Autodesk Inventor part; units mm, degrees
(part 2 of 3)
  arc A340 (-25.1328, 93.8701) -> (-24.6328, 93.3701) centre (-24.6328, 93.8701) ccw
  arc A341 (-24.6328, 100.3701) -> (-25.1328, 99.8701) centre (-24.6328, 99.8701) ccw
  arc A342 (-10.6328, 93.3701) -> (-10.1328, 93.8701) centre (-10.6328, 93.8701) ccw
  arc A343 (-10.1328, 99.8701) -> (-10.6328, 100.3701) centre (-10.6328, 99.8701) ccw
  line L344 (-25.1328, 193.8701) -> (-25.1328, 199.8701)
  line L345 (-10.1328, 193.8701) -> (-10.1328, 199.8701)
  line L346 (-24.6328, 193.3701) -> (-10.6328, 193.3701)
  line L347 (-24.6328, 200.3701) -> (-10.6328, 200.3701)
  arc A344 (-25.1328, 193.8701) -> (-24.6328, 193.3701) centre (-24.6328, 193.8701) ccw
  arc A345 (-24.6328, 200.3701) -> (-25.1328, 199.8701) centre (-24.6328, 199.8701) ccw
  arc A346 (-10.6328, 193.3701) -> (-10.1328, 193.8701) centre (-10.6328, 193.8701) ccw
  arc A347 (-10.1328, 199.8701) -> (-10.6328, 200.3701) centre (-10.6328, 199.8701) ccw
  line L348 (-26.1328, 211.8076) -> (-26.1328, 224.8076)
  line L349 (-12.1328, 211.8076) -> (-12.1328, 224.8076)
  line L350 (-25.6328, 211.3076) -> (-12.6328, 211.3076)
  line L351 (-25.6328, 225.3076) -> (-12.6328, 225.3076)
  arc A348 (-26.1328, 211.8076) -> (-25.6328, 211.3076) centre (-25.6328, 211.8076) ccw
  arc A349 (-25.6328, 225.3076) -> (-26.1328, 224.8076) centre (-25.6328, 224.8076) ccw
  arc A350 (-12.6328, 211.3076) -> (-12.1328, 211.8076) centre (-12.6328, 211.8076) ccw
  arc A351 (-12.1328, 224.8076) -> (-12.6328, 225.3076) centre (-12.6328, 224.8076) ccw
  line L352 (-26.1328, 235.6201) -> (-26.1328, 248.6201)
  line L353 (-12.1328, 235.6201) -> (-12.1328, 248.6201)
  line L354 (-25.6328, 235.1201) -> (-12.6328, 235.1201)
  line L355 (-25.6328, 249.1201) -> (-12.6328, 249.1201)
  arc A352 (-26.1328, 235.6201) -> (-25.6328, 235.1201) centre (-25.6328, 235.6201) ccw
  arc A353 (-25.6328, 249.1201) -> (-26.1328, 248.6201) centre (-25.6328, 248.6201) ccw
  arc A354 (-12.6328, 235.1201) -> (-12.1328, 235.6201) centre (-12.6328, 235.6201) ccw
  arc A355 (-12.1328, 248.6201) -> (-12.6328, 249.1201) centre (-12.6328, 248.6201) ccw
  line L356 (-26.1328, 259.4326) -> (-26.1328, 272.4326)
  line L357 (-12.1328, 259.4326) -> (-12.1328, 272.4326)
  line L358 (-25.6328, 258.9326) -> (-12.6328, 258.9326)
  line L359 (-25.6328, 272.9326) -> (-12.6328, 272.9326)
  arc A356 (-26.1328, 259.4326) -> (-25.6328, 258.9326) centre (-25.6328, 259.4326) ccw
  arc A357 (-25.6328, 272.9326) -> (-26.1328, 272.4326) centre (-25.6328, 272.4326) ccw
  arc A358 (-12.6328, 258.9326) -> (-12.1328, 259.4326) centre (-12.6328, 259.4326) ccw
  arc A359 (-12.1328, 272.4326) -> (-12.6328, 272.9326) centre (-12.6328, 272.4326) ccw
  line L360 (-26.1328, 283.2451) -> (-26.1328, 296.2451)
  line L361 (-12.1328, 283.2451) -> (-12.1328, 296.2451)
  line L362 (-25.6328, 282.7451) -> (-12.6328, 282.7451)
  line L363 (-25.6328, 296.7451) -> (-12.6328, 296.7451)
  arc A360 (-26.1328, 283.2451) -> (-25.6328, 282.7451) centre (-25.6328, 283.2451) ccw
  arc A361 (-25.6328, 296.7451) -> (-26.1328, 296.2451) centre (-25.6328, 296.2451) ccw
  arc A362 (-12.6328, 282.7451) -> (-12.1328, 283.2451) centre (-12.6328, 283.2451) ccw
  arc A363 (-12.1328, 296.2451) -> (-12.6328, 296.7451) centre (-12.6328, 296.2451) ccw
  line L364 (-26.1328, 309.4388) -> (-26.1328, 322.4388)
  line L365 (-12.1328, 309.4388) -> (-12.1328, 322.4388)
  line L366 (-25.6328, 308.9388) -> (-12.6328, 308.9388)
  line L367 (-25.6328, 322.9388) -> (-12.6328, 322.9388)
  arc A364 (-26.1328, 309.4388) -> (-25.6328, 308.9388) centre (-25.6328, 309.4388) ccw
  arc A365 (-25.6328, 322.9388) -> (-26.1328, 322.4388) centre (-25.6328, 322.4388) ccw
  arc A366 (-12.6328, 308.9388) -> (-12.1328, 309.4388) centre (-12.6328, 309.4388) ccw
  arc A367 (-12.1328, 322.4388) -> (-12.6328, 322.9388) centre (-12.6328, 322.4388) ccw
  line L368 (-26.1328, 328.4888) -> (-26.1328, 341.4888)
  line L369 (-12.1328, 328.4888) -> (-12.1328, 341.4888)
  line L370 (-25.6328, 327.9888) -> (-12.6328, 327.9888)
  line L371 (-25.6328, 341.9888) -> (-12.6328, 341.9888)
  arc A368 (-26.1328, 328.4888) -> (-25.6328, 327.9888) centre (-25.6328, 328.4888) ccw
  arc A369 (-25.6328, 341.9888) -> (-26.1328, 341.4888) centre (-25.6328, 341.4888) ccw
  arc A370 (-12.6328, 327.9888) -> (-12.1328, 328.4888) centre (-12.6328, 328.4888) ccw
  arc A371 (-12.1328, 341.4888) -> (-12.6328, 341.9888) centre (-12.6328, 341.4888) ccw
  line L372 (-26.1328, 347.5388) -> (-26.1328, 360.5388)
  line L373 (-12.1328, 347.5388) -> (-12.1328, 360.5388)
  line L374 (-25.6328, 347.0388) -> (-12.6328, 347.0388)
  line L375 (-25.6328, 361.0388) -> (-12.6328, 361.0388)
  arc A372 (-26.1328, 347.5388) -> (-25.6328, 347.0388) centre (-25.6328, 347.5388) ccw
  arc A373 (-25.6328, 361.0388) -> (-26.1328, 360.5388) centre (-25.6328, 360.5388) ccw
  arc A374 (-12.6328, 347.0388) -> (-12.1328, 347.5388) centre (-12.6328, 347.5388) ccw
  arc A375 (-12.1328, 360.5388) -> (-12.6328, 361.0388) centre (-12.6328, 360.5388) ccw
  line L376 (-9.6078, 15.9013) -> (-9.6078, 363.5638)
  line L377 (-133.4328, 15.9013) -> (-133.4328, 363.5638)
  line L378 (-9.6078, 15.9013) -> (-133.4328, 15.9013)
  line L379 (-9.6078, 363.5638) -> (-133.4328, 363.5638)
  point P0 (-68.7393, 181.4626)
sketch "Sketch1" plane through (0, 0, 0) normal (0, 1, 0) x (-1, 0, 0)
  line L0 (0, 0) -> (144.19, 0)
  line L1 (144.19, 0) -> (144.19, -379.14)
  line L2 (144.19, -379.14) -> (0, -379.14)
  line L3 (0, -379.14) -> (0, 0)
  dimension "d0" = 144.19
  dimension "d1" = 379.14
  constraints: 8 end point, 2 parallel, 1 horizontal, 1 perpendicular
  measures "d0" distance of L1.end L2.end
  measures "d1" distance of L0.end L1.end
extrude "Extrusion1" add sketch "Sketch1" along normal blind 2
sketch "Sketch3" plane through (0, 2, 0) normal (0, 1, 0) x (1, 0, 0)
  line L0 (-144.19, 0) -> (0, 0) projected
  line L1 (-144.19, 379.14) -> (-144.19, 0) projected
  line L2 (-131.665, 13.025) -> (-131.665, 26.025)
  line L3 (-117.665, 13.025) -> (-117.665, 26.025)
  line L4 (-131.165, 12.525) -> (-118.165, 12.525)
  line L5 (-131.165, 26.525) -> (-118.165, 26.525)
  arc A0 (-131.665, 13.025) -> (-131.165, 12.525) centre (-131.165, 13.025) ccw
  arc A1 (-131.165, 26.525) -> (-131.665, 26.025) centre (-131.165, 26.025) ccw
  arc A2 (-118.165, 12.525) -> (-117.665, 13.025) centre (-118.165, 13.025) ccw
  arc A3 (-117.665, 26.025) -> (-118.165, 26.525) centre (-118.165, 26.025) ccw
  line L6 (-131.665, 51.125) -> (-131.665, 64.125)
  line L7 (-117.665, 51.125) -> (-117.665, 64.125)
  line L8 (-131.165, 50.625) -> (-118.165, 50.625)
  line L9 (-131.165, 64.625) -> (-118.165, 64.625)
  arc A4 (-131.665, 51.125) -> (-131.165, 50.625) centre (-131.165, 51.125) ccw
  arc A5 (-131.165, 64.625) -> (-131.665, 64.125) centre (-131.165, 64.125) ccw
  arc A6 (-118.165, 50.625) -> (-117.665, 51.125) centre (-118.165, 51.125) ccw
  arc A7 (-117.665, 64.125) -> (-118.165, 64.625) centre (-118.165, 64.125) ccw
  line L10 (-131.665, 70.175) -> (-131.665, 83.175)
  line L11 (-117.665, 70.175) -> (-117.665, 83.175)
  line L12 (-131.165, 69.675) -> (-118.165, 69.675)
  line L13 (-131.165, 83.675) -> (-118.165, 83.675)
  arc A8 (-131.665, 70.175) -> (-131.165, 69.675) centre (-131.165, 70.175) ccw
  arc A9 (-131.165, 83.675) -> (-131.665, 83.175) centre (-131.165, 83.175) ccw
  arc A10 (-118.165, 69.675) -> (-117.665, 70.175) centre (-118.165, 70.175) ccw
  arc A11 (-117.665, 83.175) -> (-118.165, 83.675) centre (-118.165, 83.175) ccw
  line L14 (-131.665, 89.225) -> (-131.665, 102.225)
  line L15 (-117.665, 89.225) -> (-117.665, 102.225)
  line L16 (-131.165, 88.725) -> (-118.165, 88.725)
  line L17 (-131.165, 102.725) -> (-118.165, 102.725)
  arc A12 (-131.665, 89.225) -> (-131.165, 88.725) centre (-131.165, 89.225) ccw
  arc A13 (-131.165, 102.725) -> (-131.665, 102.225) centre (-131.165, 102.225) ccw
  arc A14 (-118.165, 88.725) -> (-117.665, 89.225) centre (-118.165, 89.225) ccw
  arc A15 (-117.665, 102.225) -> (-118.165, 102.725) centre (-118.165, 102.225) ccw
  line L18 (-131.665, 108.275) -> (-131.665, 121.275)
  line L19 (-117.665, 108.275) -> (-117.665, 121.275)
  line L20 (-131.165, 107.775) -> (-118.165, 107.775)
  line L21 (-131.165, 121.775) -> (-118.165, 121.775)
  arc A16 (-131.665, 108.275) -> (-131.165, 107.775) centre (-131.165, 108.275) ccw
  arc A17 (-131.165, 121.775) -> (-131.665, 121.275) centre (-131.165, 121.275) ccw
  arc A18 (-118.165, 107.775) -> (-117.665, 108.275) centre (-118.165, 108.275) ccw
  arc A19 (-117.665, 121.275) -> (-118.165, 121.775) centre (-118.165, 121.275) ccw
  line L22 (-131.665, 136.85) -> (-131.665, 149.85)
  line L23 (-117.665, 136.85) -> (-117.665, 149.85)
  line L24 (-131.165, 136.35) -> (-118.165, 136.35)
  line L25 (-131.165, 150.35) -> (-118.165, 150.35)
  arc A20 (-131.665, 136.85) -> (-131.165, 136.35) centre (-131.165, 136.85) ccw
  arc A21 (-131.165, 150.35) -> (-131.665, 149.85) centre (-131.165, 149.85) ccw
  arc A22 (-118.165, 136.35) -> (-117.665, 136.85) centre (-118.165, 136.85) ccw
  arc A23 (-117.665, 149.85) -> (-118.165, 150.35) centre (-118.165, 149.85) ccw
  line L26 (-131.665, 155.9) -> (-131.665, 168.9)
  line L27 (-117.665, 155.9) -> (-117.665, 168.9)
  line L28 (-131.165, 155.4) -> (-118.165, 155.4)
  line L29 (-131.165, 169.4) -> (-118.165, 169.4)
  arc A24 (-131.665, 155.9) -> (-131.165, 155.4) centre (-131.165, 155.9) ccw
  arc A25 (-131.165, 169.4) -> (-131.665, 168.9) centre (-131.165, 168.9) ccw
  arc A26 (-118.165, 155.4) -> (-117.665, 155.9) centre (-118.165, 155.9) ccw
  arc A27 (-117.665, 168.9) -> (-118.165, 169.4) centre (-118.165, 168.9) ccw
  line L30 (-131.665, 174.95) -> (-131.665, 187.95)
  line L31 (-117.665, 174.95) -> (-117.665, 187.95)
  line L32 (-131.165, 174.45) -> (-118.165, 174.45)
  line L33 (-131.165, 188.45) -> (-118.165, 188.45)
  arc A28 (-131.665, 174.95) -> (-131.165, 174.45) centre (-131.165, 174.95) ccw
  arc A29 (-131.165, 188.45) -> (-131.665, 187.95) centre (-131.165, 187.95) ccw
  arc A30 (-118.165, 174.45) -> (-117.665, 174.95) centre (-118.165, 174.95) ccw
  arc A31 (-117.665, 187.95) -> (-118.165, 188.45) centre (-118.165, 187.95) ccw
  line L34 (-131.665, 194) -> (-131.665, 207)
  line L35 (-117.665, 194) -> (-117.665, 207)
  line L36 (-131.165, 193.5) -> (-118.165, 193.5)
  line L37 (-131.165, 207.5) -> (-118.165, 207.5)
  arc A32 (-131.665, 194) -> (-131.165, 193.5) centre (-131.165, 194) ccw
  arc A33 (-131.165, 207.5) -> (-131.665, 207) centre (-131.165, 207) ccw
  arc A34 (-118.165, 193.5) -> (-117.665, 194) centre (-118.165, 194) ccw
  arc A35 (-117.665, 207) -> (-118.165, 207.5) centre (-118.165, 207) ccw
  line L38 (-131.665, 222.575) -> (-131.665, 235.575)
  line L39 (-117.665, 222.575) -> (-117.665, 235.575)
  line L40 (-131.165, 222.075) -> (-118.165, 222.075)
  line L41 (-131.165, 236.075) -> (-118.165, 236.075)
  arc A36 (-131.665, 222.575) -> (-131.165, 222.075) centre (-131.165, 222.575) ccw
  arc A37 (-131.165, 236.075) -> (-131.665, 235.575) centre (-131.165, 235.575) ccw
  arc A38 (-118.165, 222.075) -> (-117.665, 222.575) centre (-118.165, 222.575) ccw
  arc A39 (-117.665, 235.575) -> (-118.165, 236.075) centre (-118.165, 235.575) ccw
  line L42 (-131.665, 241.625) -> (-131.665, 254.625)
  line L43 (-117.665, 241.625) -> (-117.665, 254.625)
  line L44 (-131.165, 241.125) -> (-118.165, 241.125)
  line L45 (-131.165, 255.125) -> (-118.165, 255.125)
  arc A40 (-131.665, 241.625) -> (-131.165, 241.125) centre (-131.165, 241.625) ccw
  arc A41 (-131.165, 255.125) -> (-131.665, 254.625) centre (-131.165, 254.625) ccw
  arc A42 (-118.165, 241.125) -> (-117.665, 241.625) centre (-118.165, 241.625) ccw
  arc A43 (-117.665, 254.625) -> (-118.165, 255.125) centre (-118.165, 254.625) ccw
  line L46 (-131.665, 260.675) -> (-131.665, 273.675)
  line L47 (-117.665, 260.675) -> (-117.665, 273.675)
  line L48 (-131.165, 260.175) -> (-118.165, 260.175)
  line L49 (-131.165, 274.175) -> (-118.165, 274.175)
  arc A44 (-131.665, 260.675) -> (-131.165, 260.175) centre (-131.165, 260.675) ccw
  arc A45 (-131.165, 274.175) -> (-131.665, 273.675) centre (-131.165, 273.675) ccw
  arc A46 (-118.165, 260.175) -> (-117.665, 260.675) centre (-118.165, 260.675) ccw
  arc A47 (-117.665, 273.675) -> (-118.165, 274.175) centre (-118.165, 273.675) ccw
  line L50 (-131.665, 279.725) -> (-131.665, 292.725)
  line L51 (-117.665, 279.725) -> (-117.665, 292.725)
  line L52 (-131.165, 279.225) -> (-118.165, 279.225)
  line L53 (-131.165, 293.225) -> (-118.165, 293.225)
  arc A48 (-131.665, 279.725) -> (-131.165, 279.225) centre (-131.165, 279.725) ccw
  arc A49 (-131.165, 293.225) -> (-131.665, 292.725) centre (-131.165, 292.725) ccw
  arc A50 (-118.165, 279.225) -> (-117.665, 279.725) centre (-118.165, 279.725) ccw
  arc A51 (-117.665, 292.725) -> (-118.165, 293.225) centre (-118.165, 292.725) ccw
  line L54 (-103.09, 13.025) -> (-103.09, 26.025)
  line L55 (-89.09, 13.025) -> (-89.09, 26.025)
  line L56 (-102.59, 12.525) -> (-89.59, 12.525)
  line L57 (-102.59, 26.525) -> (-89.59, 26.525)
  arc A52 (-103.09, 13.025) -> (-102.59, 12.525) centre (-102.59, 13.025) ccw
  arc A53 (-102.59, 26.525) -> (-103.09, 26.025) centre (-102.59, 26.025) ccw
  arc A54 (-89.59, 12.525) -> (-89.09, 13.025) centre (-89.59, 13.025) ccw
  arc A55 (-89.09, 26.025) -> (-89.59, 26.525) centre (-89.59, 26.025) ccw
  line L58 (-103.09, 32.075) -> (-103.09, 45.075)
  line L59 (-89.09, 32.075) -> (-89.09, 45.075)
  line L60 (-102.59, 31.575) -> (-89.59, 31.575)
  line L61 (-102.59, 45.575) -> (-89.59, 45.575)
  arc A56 (-103.09, 32.075) -> (-102.59, 31.575) centre (-102.59, 32.075) ccw
  arc A57 (-102.59, 45.575) -> (-103.09, 45.075) centre (-102.59, 45.075) ccw
  arc A58 (-89.59, 31.575) -> (-89.09, 32.075) centre (-89.59, 32.075) ccw
  arc A59 (-89.09, 45.075) -> (-89.59, 45.575) centre (-89.59, 45.075) ccw
  line L62 (-103.09, 51.125) -> (-103.09, 64.125)
  line L63 (-89.09, 51.125) -> (-89.09, 64.125)
  line L64 (-102.59, 50.625) -> (-89.59, 50.625)
  line L65 (-102.59, 64.625) -> (-89.59, 64.625)
  arc A60 (-103.09, 51.125) -> (-102.59, 50.625) centre (-102.59, 51.125) ccw
  arc A61 (-102.59, 64.625) -> (-103.09, 64.125) centre (-102.59, 64.125) ccw
  arc A62 (-89.59, 50.625) -> (-89.09, 51.125) centre (-89.59, 51.125) ccw
  arc A63 (-89.09, 64.125) -> (-89.59, 64.625) centre (-89.59, 64.125) ccw
  line L66 (-103.09, 70.175) -> (-103.09, 83.175)
  line L67 (-89.09, 70.175) -> (-89.09, 83.175)
  line L68 (-102.59, 69.675) -> (-89.59, 69.675)
  line L69 (-102.59, 83.675) -> (-89.59, 83.675)
  arc A64 (-103.09, 70.175) -> (-102.59, 69.675) centre (-102.59, 70.175) ccw
  arc A65 (-102.59, 83.675) -> (-103.09, 83.175) centre (-102.59, 83.175) ccw
  arc A66 (-89.59, 69.675) -> (-89.09, 70.175) centre (-89.59, 70.175) ccw
  arc A67 (-89.09, 83.175) -> (-89.59, 83.675) centre (-89.59, 83.175) ccw
  line L70 (-103.09, 89.225) -> (-103.09, 102.225)
  line L71 (-89.09, 89.225) -> (-89.09, 102.225)
  line L72 (-102.59, 88.725) -> (-89.59, 88.725)
  line L73 (-102.59, 102.725) -> (-89.59, 102.725)
  arc A68 (-103.09, 89.225) -> (-102.59, 88.725) centre (-102.59, 89.225) ccw
  arc A69 (-102.59, 102.725) -> (-103.09, 102.225) centre (-102.59, 102.225) ccw
  arc A70 (-89.59, 88.725) -> (-89.09, 89.225) centre (-89.59, 89.225) ccw
  arc A71 (-89.09, 102.225) -> (-89.59, 102.725) centre (-89.59, 102.225) ccw
  line L74 (-103.09, 108.275) -> (-103.09, 121.275)
  line L75 (-89.09, 108.275) -> (-89.09, 121.275)
  line L76 (-102.59, 107.775) -> (-89.59, 107.775)
  line L77 (-102.59, 121.775) -> (-89.59, 121.775)
  arc A72 (-103.09, 108.275) -> (-102.59, 107.775) centre (-102.59, 108.275) ccw
  arc A73 (-102.59, 121.775) -> (-103.09, 121.275) centre (-102.59, 121.275) ccw
  arc A74 (-89.59, 107.775) -> (-89.09, 108.275) centre (-89.59, 108.275) ccw
  arc A75 (-89.09, 121.275) -> (-89.59, 121.775) centre (-89.59, 121.275) ccw
  line L78 (-103.09, 127.325) -> (-103.09, 140.325)
  line L79 (-89.09, 127.325) -> (-89.09, 140.325)
  line L80 (-102.59, 126.825) -> (-89.59, 126.825)
  line L81 (-102.59, 140.825) -> (-89.59, 140.825)
  arc A76 (-103.09, 127.325) -> (-102.59, 126.825) centre (-102.59, 127.325) ccw
  arc A77 (-102.59, 140.825) -> (-103.09, 140.325) centre (-102.59, 140.325) ccw
  arc A78 (-89.59, 126.825) -> (-89.09, 127.325) centre (-89.59, 127.325) ccw
  arc A79 (-89.09, 140.325) -> (-89.59, 140.825) centre (-89.59, 140.325) ccw
  line L82 (-103.09, 146.375) -> (-103.09, 159.375)
  line L83 (-89.09, 146.375) -> (-89.09, 159.375)
  line L84 (-102.59, 145.875) -> (-89.59, 145.875)
  line L85 (-102.59, 159.875) -> (-89.59, 159.875)
  arc A80 (-103.09, 146.375) -> (-102.59, 145.875) centre (-102.59, 146.375) ccw
  arc A81 (-102.59, 159.875) -> (-103.09, 159.375) centre (-102.59, 159.375) ccw
  arc A82 (-89.59, 145.875) -> (-89.09, 146.375) centre (-89.59, 146.375) ccw
  arc A83 (-89.09, 159.375) -> (-89.59, 159.875) centre (-89.59, 159.375) ccw
  line L86 (-103.09, 165.425) -> (-103.09, 178.425)
  line L87 (-89.09, 165.425) -> (-89.09, 178.425)
  line L88 (-102.59, 164.925) -> (-89.59, 164.925)
  line L89 (-102.59, 178.925) -> (-89.59, 178.925)
  arc A84 (-103.09, 165.425) -> (-102.59, 164.925) centre (-102.59, 165.425) ccw
  arc A85 (-102.59, 178.925) -> (-103.09, 178.425) centre (-102.59, 178.425) ccw
  arc A86 (-89.59, 164.925) -> (-89.09, 165.425) centre (-89.59, 165.425) ccw
  arc A87 (-89.09, 178.425) -> (-89.59, 178.925) centre (-89.59, 178.425) ccw
  line L90 (-103.09, 184.475) -> (-103.09, 197.475)
  line L91 (-89.09, 184.475) -> (-89.09, 197.475)
  line L92 (-102.59, 183.975) -> (-89.59, 183.975)
  line L93 (-102.59, 197.975) -> (-89.59, 197.975)
  arc A88 (-103.09, 184.475) -> (-102.59, 183.975) centre (-102.59, 184.475) ccw
  arc A89 (-102.59, 197.975) -> (-103.09, 197.475) centre (-102.59, 197.475) ccw
  arc A90 (-89.59, 183.975) -> (-89.09, 184.475) centre (-89.59, 184.475) ccw
  arc A91 (-89.09, 197.475) -> (-89.59, 197.975) centre (-89.59, 197.475) ccw
  line L94 (-103.09, 203.525) -> (-103.09, 216.525)
  line L95 (-89.09, 203.525) -> (-89.09, 216.525)
  line L96 (-102.59, 203.025) -> (-89.59, 203.025)
  line L97 (-102.59, 217.025) -> (-89.59, 217.025)
  arc A92 (-103.09, 203.525) -> (-102.59, 203.025) centre (-102.59, 203.525) ccw
  arc A93 (-102.59, 217.025) -> (-103.09, 216.525) centre (-102.59, 216.525) ccw
  arc A94 (-89.59, 203.025) -> (-89.09, 203.525) centre (-89.59, 203.525) ccw
  arc A95 (-89.09, 216.525) -> (-89.59, 217.025) centre (-89.59, 216.525) ccw
  line L98 (-103.09, 222.575) -> (-103.09, 235.575)
  line L99 (-89.09, 222.575) -> (-89.09, 235.575)
  line L100 (-102.59, 222.075) -> (-89.59, 222.075)
  line L101 (-102.59, 236.075) -> (-89.59, 236.075)
  arc A96 (-103.09, 222.575) -> (-102.59, 222.075) centre (-102.59, 222.575) ccw
  arc A97 (-102.59, 236.075) -> (-103.09, 235.575) centre (-102.59, 235.575) ccw
  arc A98 (-89.59, 222.075) -> (-89.09, 222.575) centre (-89.59, 222.575) ccw
  arc A99 (-89.09, 235.575) -> (-89.59, 236.075) centre (-89.59, 235.575) ccw
  line L102 (-103.09, 241.625) -> (-103.09, 254.625)
  line L103 (-89.09, 241.625) -> (-89.09, 254.625)
  line L104 (-102.59, 241.125) -> (-89.59, 241.125)
  line L105 (-102.59, 255.125) -> (-89.59, 255.125)
  arc A100 (-103.09, 241.625) -> (-102.59, 241.125) centre (-102.59, 241.625) ccw
  arc A101 (-102.59, 255.125) -> (-103.09, 254.625) centre (-102.59, 254.625) ccw
  arc A102 (-89.59, 241.125) -> (-89.09, 241.625) centre (-89.59, 241.625) ccw
  arc A103 (-89.09, 254.625) -> (-89.59, 255.125) centre (-89.59, 254.625) ccw
  line L106 (-103.09, 270.2) -> (-103.09, 283.2)
  line L107 (-89.09, 270.2) -> (-89.09, 283.2)
  line L108 (-102.59, 269.7) -> (-89.59, 269.7)
  line L109 (-102.59, 283.7) -> (-89.59, 283.7)
  arc A104 (-103.09, 270.2) -> (-102.59, 269.7) centre (-102.59, 270.2) ccw
  arc A105 (-102.59, 283.7) -> (-103.09, 283.2) centre (-102.59, 283.2) ccw
  arc A106 (-89.59, 269.7) -> (-89.09, 270.2) centre (-89.59, 270.2) ccw
  arc A107 (-89.09, 283.2) -> (-89.59, 283.7) centre (-89.59, 283.2) ccw
  line L110 (-102.09, 261.762) -> (-102.09, 267.762)
  line L111 (-87.09, 261.762) -> (-87.09, 267.762)
  line L112 (-101.59, 261.262) -> (-87.59, 261.262)
  line L113 (-101.59, 268.262) -> (-87.59, 268.262)
  arc A108 (-102.09, 261.762) -> (-101.59, 261.262) centre (-101.59, 261.762) ccw
  arc A109 (-101.59, 268.262) -> (-102.09, 267.762) centre (-101.59, 267.762) ccw
  arc A110 (-87.59, 261.262) -> (-87.09, 261.762) centre (-87.59, 261.762) ccw
  arc A111 (-87.09, 267.762) -> (-87.59, 268.262) centre (-87.59, 267.762) ccw
  line L114 (-102.09, 285.638) -> (-102.09, 291.638)
  line L115 (-87.09, 285.638) -> (-87.09, 291.638)
  line L116 (-101.59, 285.138) -> (-87.59, 285.138)
  line L117 (-101.59, 292.138) -> (-87.59, 292.138)
  arc A112 (-102.09, 285.638) -> (-101.59, 285.138) centre (-101.59, 285.638) ccw
  arc A113 (-101.59, 292.138) -> (-102.09, 291.638) centre (-101.59, 291.638) ccw
  arc A114 (-87.59, 285.138) -> (-87.09, 285.638) centre (-87.59, 285.638) ccw
  arc A115 (-87.09, 291.638) -> (-87.59, 292.138) centre (-87.59, 291.638) ccw
  line L118 (-103.09, 303.5375) -> (-103.09, 316.5375)
  line L119 (-89.09, 303.5375) -> (-89.09, 316.5375)
  line L120 (-102.59, 303.0375) -> (-89.59, 303.0375)
  line L121 (-102.59, 317.0375) -> (-89.59, 317.0375)
  arc A116 (-103.09, 303.5375) -> (-102.59, 303.0375) centre (-102.59, 303.5375) ccw
  arc A117 (-102.59, 317.0375) -> (-103.09, 316.5375) centre (-102.59, 316.5375) ccw
  arc A118 (-89.59, 303.0375) -> (-89.09, 303.5375) centre (-89.59, 303.5375) ccw
  arc A119 (-89.09, 316.5375) -> (-89.59, 317.0375) centre (-89.59, 316.5375) ccw
  line L122 (-103.09, 322.5875) -> (-103.09, 335.5875)
  line L123 (-89.09, 322.5875) -> (-89.09, 335.5875)
  line L124 (-102.59, 322.0875) -> (-89.59, 322.0875)
  line L125 (-102.59, 336.0875) -> (-89.59, 336.0875)
  arc A120 (-103.09, 322.5875) -> (-102.59, 322.0875) centre (-102.59, 322.5875) ccw
  arc A121 (-102.59, 336.0875) -> (-103.09, 335.5875) centre (-102.59, 335.5875) ccw
  arc A122 (-89.59, 322.0875) -> (-89.09, 322.5875) centre (-89.59, 322.5875) ccw
  arc A123 (-89.09, 335.5875) -> (-89.59, 336.0875) centre (-89.59, 335.5875) ccw
  line L126 (-103.09, 341.6375) -> (-103.09, 354.6375)
  line L127 (-89.09, 341.6375) -> (-89.09, 354.6375)
  line L128 (-102.59, 341.1375) -> (-89.59, 341.1375)
  line L129 (-102.59, 355.1375) -> (-89.59, 355.1375)
  arc A124 (-103.09, 341.6375) -> (-102.59, 341.1375) centre (-102.59, 341.6375) ccw
  arc A125 (-102.59, 355.1375) -> (-103.09, 354.6375) centre (-102.59, 354.6375) ccw
  arc A126 (-89.59, 341.1375) -> (-89.09, 341.6375) centre (-89.59, 341.6375) ccw
  arc A127 (-89.09, 354.6375) -> (-89.59, 355.1375) centre (-89.59, 354.6375) ccw
  line L130 (-84.04, 17.7875) -> (-84.04, 30.7875)
  line L131 (-70.04, 17.7875) -> (-70.04, 30.7875)
  line L132 (-83.54, 17.2875) -> (-70.54, 17.2875)
  line L133 (-83.54, 31.2875) -> (-70.54, 31.2875)
  arc A128 (-84.04, 17.7875) -> (-83.54, 17.2875) centre (-83.54, 17.7875) ccw
  arc A129 (-83.54, 31.2875) -> (-84.04, 30.7875) centre (-83.54, 30.7875) ccw
  arc A130 (-70.54, 17.2875) -> (-70.04, 17.7875) centre (-70.54, 17.7875) ccw
  arc A131 (-70.04, 30.7875) -> (-70.54, 31.2875) centre (-70.54, 30.7875) ccw
  line L134 (-84.04, 41.6) -> (-84.04, 54.6)
  line L135 (-70.04, 41.6) -> (-70.04, 54.6)
  line L136 (-83.54, 41.1) -> (-70.54, 41.1)
  line L137 (-83.54, 55.1) -> (-70.54, 55.1)
  arc A132 (-84.04, 41.6) -> (-83.54, 41.1) centre (-83.54, 41.6) ccw
  arc A133 (-83.54, 55.1) -> (-84.04, 54.6) centre (-83.54, 54.6) ccw
  arc A134 (-70.54, 41.1) -> (-70.04, 41.6) centre (-70.54, 41.6) ccw
  arc A135 (-70.04, 54.6) -> (-70.54, 55.1) centre (-70.54, 54.6) ccw
  line L138 (-84.04, 60.65) -> (-84.04, 73.65)
  line L139 (-70.04, 60.65) -> (-70.04, 73.65)
  line L140 (-83.54, 60.15) -> (-70.54, 60.15)
  line L141 (-83.54, 74.15) -> (-70.54, 74.15)
  arc A136 (-84.04, 60.65) -> (-83.54, 60.15) centre (-83.54, 60.65) ccw
  arc A137 (-83.54, 74.15) -> (-84.04, 73.65) centre (-83.54, 73.65) ccw
  arc A138 (-70.54, 60.15) -> (-70.04, 60.65) centre (-70.54, 60.65) ccw
  arc A139 (-70.04, 73.65) -> (-70.54, 74.15) centre (-70.54, 73.65) ccw
  line L142 (-84.04, 79.7) -> (-84.04, 92.7)
  line L143 (-70.04, 79.7) -> (-70.04, 92.7)
  line L144 (-83.54, 79.2) -> (-70.54, 79.2)
  line L145 (-83.54, 93.2) -> (-70.54, 93.2)
  arc A140 (-84.04, 79.7) -> (-83.54, 79.2) centre (-83.54, 79.7) ccw
  arc A141 (-83.54, 93.2) -> (-84.04, 92.7) centre (-83.54, 92.7) ccw
  arc A142 (-70.54, 79.2) -> (-70.04, 79.7) centre (-70.54, 79.7) ccw
  arc A143 (-70.04, 92.7) -> (-70.54, 93.2) centre (-70.54, 92.7) ccw
  line L146 (-84.04, 98.75) -> (-84.04, 111.75)
  line L147 (-70.04, 98.75) -> (-70.04, 111.75)
  line L148 (-83.54, 98.25) -> (-70.54, 98.25)
  line L149 (-83.54, 112.25) -> (-70.54, 112.25)
  arc A144 (-84.04, 98.75) -> (-83.54, 98.25) centre (-83.54, 98.75) ccw
  arc A145 (-83.54, 112.25) -> (-84.04, 111.75) centre (-83.54, 111.75) ccw
  arc A146 (-70.54, 98.25) -> (-70.04, 98.75) centre (-70.54, 98.75) ccw
  arc A147 (-70.04, 111.75) -> (-70.54, 112.25) centre (-70.54, 111.75) ccw
  line L150 (-84.04, 117.8) -> (-84.04, 130.8)
  line L151 (-70.04, 117.8) -> (-70.04, 130.8)
  line L152 (-83.54, 117.3) -> (-70.54, 117.3)
  line L153 (-83.54, 131.3) -> (-70.54, 131.3)
  arc A148 (-84.04, 117.8) -> (-83.54, 117.3) centre (-83.54, 117.8) ccw
  arc A149 (-83.54, 131.3) -> (-84.04, 130.8) centre (-83.54, 130.8) ccw
  arc A150 (-70.54, 117.3) -> (-70.04, 117.8) centre (-70.54, 117.8) ccw
  arc A151 (-70.04, 130.8) -> (-70.54, 131.3) centre (-70.54, 130.8) ccw
  line L154 (-84.04, 136.85) -> (-84.04, 149.85)
  line L155 (-70.04, 136.85) -> (-70.04, 149.85)
  line L156 (-83.54, 136.35) -> (-70.54, 136.35)
  line L157 (-83.54, 150.35) -> (-70.54, 150.35)
  arc A152 (-84.04, 136.85) -> (-83.54, 136.35) centre (-83.54, 136.85) ccw
  arc A153 (-83.54, 150.35) -> (-84.04, 149.85) centre (-83.54, 149.85) ccw
  arc A154 (-70.54, 136.35) -> (-70.04, 136.85) centre (-70.54, 136.85) ccw
  arc A155 (-70.04, 149.85) -> (-70.54, 150.35) centre (-70.54, 149.85) ccw
  line L158 (-84.04, 155.9) -> (-84.04, 168.9)
  line L159 (-70.04, 155.9) -> (-70.04, 168.9)
  line L160 (-83.54, 155.4) -> (-70.54, 155.4)
  line L161 (-83.54, 169.4) -> (-70.54, 169.4)
  arc A156 (-84.04, 155.9) -> (-83.54, 155.4) centre (-83.54, 155.9) ccw
  arc A157 (-83.54, 169.4) -> (-84.04, 168.9) centre (-83.54, 168.9) ccw
  arc A158 (-70.54, 155.4) -> (-70.04, 155.9) centre (-70.54, 155.9) ccw
  arc A159 (-70.04, 168.9) -> (-70.54, 169.4) centre (-70.54, 168.9) ccw
  line L162 (-84.04, 174.95) -> (-84.04, 187.95)
  line L163 (-70.04, 174.95) -> (-70.04, 187.95)
  line L164 (-83.54, 174.45) -> (-70.54, 174.45)
  line L165 (-83.54, 188.45) -> (-70.54, 188.45)
  arc A160 (-84.04, 174.95) -> (-83.54, 174.45) centre (-83.54, 174.95) ccw
  arc A161 (-83.54, 188.45) -> (-84.04, 187.95) centre (-83.54, 187.95) ccw
  arc A162 (-70.54, 174.45) -> (-70.04, 174.95) centre (-70.54, 174.95) ccw
  arc A163 (-70.04, 187.95) -> (-70.54, 188.45) centre (-70.54, 187.95) ccw
  line L166 (-84.04, 194) -> (-84.04, 207)
  line L167 (-70.04, 194) -> (-70.04, 207)
  line L168 (-83.54, 193.5) -> (-70.54, 193.5)
  line L169 (-83.54, 207.5) -> (-70.54, 207.5)
  arc A164 (-84.04, 194) -> (-83.54, 193.5) centre (-83.54, 194) ccw
  arc A165 (-83.54, 207.5) -> (-84.04, 207) centre (-83.54, 207) ccw
  arc A166 (-70.54, 193.5) -> (-70.04, 194) centre (-70.54, 194) ccw
  arc A167 (-70.04, 207) -> (-70.54, 207.5) centre (-70.54, 207) ccw
  line L170 (-84.04, 213.05) -> (-84.04, 226.05)
  line L171 (-70.04, 213.05) -> (-70.04, 226.05)
  line L172 (-83.54, 212.55) -> (-70.54, 212.55)
  line L173 (-83.54, 226.55) -> (-70.54, 226.55)
  arc A168 (-84.04, 213.05) -> (-83.54, 212.55) centre (-83.54, 213.05) ccw
  arc A169 (-83.54, 226.55) -> (-84.04, 226.05) centre (-83.54, 226.05) ccw
  arc A170 (-70.54, 212.55) -> (-70.04, 213.05) centre (-70.54, 213.05) ccw
  arc A171 (-70.04, 226.05) -> (-70.54, 226.55) centre (-70.54, 226.05) ccw
  line L174 (-84.04, 232.1) -> (-84.04, 245.1)
  line L175 (-70.04, 232.1) -> (-70.04, 245.1)
  line L176 (-83.54, 231.6) -> (-70.54, 231.6)
  line L177 (-83.54, 245.6) -> (-70.54, 245.6)
  arc A172 (-84.04, 232.1) -> (-83.54, 231.6) centre (-83.54, 232.1) ccw
  arc A173 (-83.54, 245.6) -> (-84.04, 245.1) centre (-83.54, 245.1) ccw
  arc A174 (-70.54, 231.6) -> (-70.04, 232.1) centre (-70.54, 232.1) ccw
  arc A175 (-70.04, 245.1) -> (-70.54, 245.6) centre (-70.54, 245.1) ccw
  line L178 (-84.04, 251.15) -> (-84.04, 264.15)
  line L179 (-70.04, 251.15) -> (-70.04, 264.15)
  line L180 (-83.54, 250.65) -> (-70.54, 250.65)
  line L181 (-83.54, 264.65) -> (-70.54, 264.65)
  arc A176 (-84.04, 251.15) -> (-83.54, 250.65) centre (-83.54, 251.15) ccw
  arc A177 (-83.54, 264.65) -> (-84.04, 264.15) centre (-83.54, 264.15) ccw
  arc A178 (-70.54, 250.65) -> (-70.04, 251.15) centre (-70.54, 251.15) ccw
  arc A179 (-70.04, 264.15) -> (-70.54, 264.65) centre (-70.54, 264.15) ccw
  line L182 (-84.04, 274.9625) -> (-84.04, 287.9625)
  line L183 (-70.04, 274.9625) -> (-70.04, 287.9625)
  line L184 (-83.54, 274.4625) -> (-70.54, 274.4625)
  line L185 (-83.54, 288.4625) -> (-70.54, 288.4625)
  arc A180 (-84.04, 274.9625) -> (-83.54, 274.4625) centre (-83.54, 274.9625) ccw
  arc A181 (-83.54, 288.4625) -> (-84.04, 287.9625) centre (-83.54, 287.9625) ccw
  arc A182 (-70.54, 274.4625) -> (-70.04, 274.9625) centre (-70.54, 274.9625) ccw
  arc A183 (-70.04, 287.9625) -> (-70.54, 288.4625) centre (-70.54, 287.9625) ccw
  line L186 (-84.04, 303.5375) -> (-84.04, 316.5375)
  line L187 (-70.04, 303.5375) -> (-70.04, 316.5375)
  line L188 (-83.54, 303.0375) -> (-70.54, 303.0375)
  line L189 (-83.54, 317.0375) -> (-70.54, 317.0375)
  arc A184 (-84.04, 303.5375) -> (-83.54, 303.0375) centre (-83.54, 303.5375) ccw
  arc A185 (-83.54, 317.0375) -> (-84.04, 316.5375) centre (-83.54, 316.5375) ccw
  arc A186 (-70.54, 303.0375) -> (-70.04, 303.5375) centre (-70.54, 303.5375) ccw
  arc A187 (-70.04, 316.5375) -> (-70.54, 317.0375) centre (-70.54, 316.5375) ccw
  line L190 (-84.04, 322.5875) -> (-84.04, 335.5875)
  line L191 (-70.04, 322.5875) -> (-70.04, 335.5875)
  line L192 (-83.54, 322.0875) -> (-70.54, 322.0875)
  line L193 (-83.54, 336.0875) -> (-70.54, 336.0875)
  arc A188 (-84.04, 322.5875) -> (-83.54, 322.0875) centre (-83.54, 322.5875) ccw
  arc A189 (-83.54, 336.0875) -> (-84.04, 335.5875) centre (-83.54, 335.5875) ccw
  arc A190 (-70.54, 322.0875) -> (-70.04, 322.5875) centre (-70.54, 322.5875) ccw
  arc A191 (-70.04, 335.5875) -> (-70.54, 336.0875) centre (-70.54, 335.5875) ccw
  line L194 (-84.04, 341.6375) -> (-84.04, 354.6375)
  line L195 (-70.04, 341.6375) -> (-70.04, 354.6375)
  line L196 (-83.54, 341.1375) -> (-70.54, 341.1375)
  line L197 (-83.54, 355.1375) -> (-70.54, 355.1375)
  arc A192 (-84.04, 341.6375) -> (-83.54, 341.1375) centre (-83.54, 341.6375) ccw
  arc A193 (-83.54, 355.1375) -> (-84.04, 354.6375) centre (-83.54, 354.6375) ccw
  arc A194 (-70.54, 341.1375) -> (-70.04, 341.6375) centre (-70.54, 341.6375) ccw
  arc A195 (-70.04, 354.6375) -> (-70.54, 355.1375) centre (-70.54, 354.6375) ccw
  line L198 (-64.99, 20.1688) -> (-64.99, 33.1688)
  line L199 (-50.99, 20.1688) -> (-50.99, 33.1688)
  line L200 (-64.49, 19.6687) -> (-51.49, 19.6688)
  line L201 (-64.49, 33.6688) -> (-51.49, 33.6688)
  arc A196 (-64.99, 20.1688) -> (-64.49, 19.6688) centre (-64.49, 20.1687) ccw
  arc A197 (-64.49, 33.6688) -> (-64.99, 33.1688) centre (-64.49, 33.1688) ccw
  arc A198 (-51.49, 19.6687) -> (-50.99, 20.1688) centre (-51.49, 20.1688) ccw
  arc A199 (-50.99, 33.1688) -> (-51.49, 33.6688) centre (-51.49, 33.1688) ccw
  line L202 (-64.99, 46.3625) -> (-64.99, 59.3625)
  line L203 (-50.99, 46.3625) -> (-50.99, 59.3625)
  line L204 (-64.49, 45.8625) -> (-51.49, 45.8625)
  line L205 (-64.49, 59.8625) -> (-51.49, 59.8625)
  arc A200 (-64.99, 46.3625) -> (-64.49, 45.8625) centre (-64.49, 46.3625) ccw
  arc A201 (-64.49, 59.8625) -> (-64.99, 59.3625) centre (-64.49, 59.3625) ccw
  arc A202 (-51.49, 45.8625) -> (-50.99, 46.3625) centre (-51.49, 46.3625) ccw
  arc A203 (-50.99, 59.3625) -> (-51.49, 59.8625) centre (-51.49, 59.3625) ccw
  line L206 (-64.99, 65.4125) -> (-64.99, 78.4125)
  line L207 (-50.99, 65.4125) -> (-50.99, 78.4125)
  line L208 (-64.49, 64.9125) -> (-51.49, 64.9125)
  line L209 (-64.49, 78.9125) -> (-51.49, 78.9125)
  arc A204 (-64.99, 65.4125) -> (-64.49, 64.9125) centre (-64.49, 65.4125) ccw
  arc A205 (-64.49, 78.9125) -> (-64.99, 78.4125) centre (-64.49, 78.4125) ccw
  arc A206 (-51.49, 64.9125) -> (-50.99, 65.4125) centre (-51.49, 65.4125) ccw
  arc A207 (-50.99, 78.4125) -> (-51.49, 78.9125) centre (-51.49, 78.4125) ccw
  line L210 (-64.99, 84.4625) -> (-64.99, 97.4625)
  line L211 (-50.99, 84.4625) -> (-50.99, 97.4625)
  line L212 (-64.49, 83.9625) -> (-51.49, 83.9625)
  line L213 (-64.49, 97.9625) -> (-51.49, 97.9625)
  arc A208 (-64.99, 84.4625) -> (-64.49, 83.9625) centre (-64.49, 84.4625) ccw
  arc A209 (-64.49, 97.9625) -> (-64.99, 97.4625) centre (-64.49, 97.4625) ccw
  arc A210 (-51.49, 83.9625) -> (-50.99, 84.4625) centre (-51.49, 84.4625) ccw
  arc A211 (-50.99, 97.4625) -> (-51.49, 97.9625) centre (-51.49, 97.4625) ccw
  line L214 (-64.99, 103.5125) -> (-64.99, 116.5125)
  line L215 (-50.99, 103.5125) -> (-50.99, 116.5125)
  line L216 (-64.49, 103.0125) -> (-51.49, 103.0125)
  line L217 (-64.49, 117.0125) -> (-51.49, 117.0125)
  arc A212 (-64.99, 103.5125) -> (-64.49, 103.0125) centre (-64.49, 103.5125) ccw
  arc A213 (-64.49, 117.0125) -> (-64.99, 116.5125) centre (-64.49, 116.5125) ccw
  arc A214 (-51.49, 103.0125) -> (-50.99, 103.5125) centre (-51.49, 103.5125) ccw
  arc A215 (-50.99, 116.5125) -> (-51.49, 117.0125) centre (-51.49, 116.5125) ccw
  line L218 (-64.99, 122.5625) -> (-64.99, 135.5625)
  line L219 (-50.99, 122.5625) -> (-50.99, 135.5625)
  line L220 (-64.49, 122.0625) -> (-51.49, 122.0625)
  line L221 (-64.49, 136.0625) -> (-51.49, 136.0625)
  arc A216 (-64.99, 122.5625) -> (-64.49, 122.0625) centre (-64.49, 122.5625) ccw
  arc A217 (-64.49, 136.0625) -> (-64.99, 135.5625) centre (-64.49, 135.5625) ccw
  arc A218 (-51.49, 122.0625) -> (-50.99, 122.5625) centre (-51.49, 122.5625) ccw
  arc A219 (-50.99, 135.5625) -> (-51.49, 136.0625) centre (-51.49, 135.5625) ccw
  line L222 (-64.99, 141.6125) -> (-64.99, 154.6125)
  line L223 (-50.99, 141.6125) -> (-50.99, 154.6125)
  line L224 (-64.49, 141.1125) -> (-51.49, 141.1125)
  line L225 (-64.49, 155.1125) -> (-51.49, 155.1125)
  arc A220 (-64.99, 141.6125) -> (-64.49, 141.1125) centre (-64.49, 141.6125) ccw
  arc A221 (-64.49, 155.1125) -> (-64.99, 154.6125) centre (-64.49, 154.6125) ccw
  arc A222 (-51.49, 141.1125) -> (-50.99, 141.6125) centre (-51.49, 141.6125) ccw
  arc A223 (-50.99, 154.6125) -> (-51.49, 155.1125) centre (-51.49, 154.6125) ccw
  line L226 (-64.99, 160.6625) -> (-64.99, 173.6625)
  line L227 (-50.99, 160.6625) -> (-50.99, 173.6625)
  line L228 (-64.49, 160.1625) -> (-51.49, 160.1625)
  line L229 (-64.49, 174.1625) -> (-51.49, 174.1625)
  arc A224 (-64.99, 160.6625) -> (-64.49, 160.1625) centre (-64.49, 160.6625) ccw
  arc A225 (-64.49, 174.1625) -> (-64.99, 173.6625) centre (-64.49, 173.6625) ccw
  arc A226 (-51.49, 160.1625) -> (-50.99, 160.6625) centre (-51.49, 160.6625) ccw
  arc A227 (-50.99, 173.6625) -> (-51.49, 174.1625) centre (-51.49, 173.6625) ccw
  line L230 (-64.99, 179.7125) -> (-64.99, 192.7125)
  line L231 (-50.99, 179.7125) -> (-50.99, 192.7125)
  line L232 (-64.49, 179.2125) -> (-51.49, 179.2125)
  line L233 (-64.49, 193.2125) -> (-51.49, 193.2125)
  arc A228 (-64.99, 179.7125) -> (-64.49, 179.2125) centre (-64.49, 179.7125) ccw
  arc A229 (-64.49, 193.2125) -> (-64.99, 192.7125) centre (-64.49, 192.7125) ccw
  arc A230 (-51.49, 179.2125) -> (-50.99, 179.7125) centre (-51.49, 179.7125) ccw
  arc A231 (-50.99, 192.7125) -> (-51.49, 193.2125) centre (-51.49, 192.7125) ccw
  line L234 (-64.99, 198.7625) -> (-64.99, 211.7625)
  line L235 (-50.99, 198.7625) -> (-50.99, 211.7625)
  line L236 (-64.49, 198.2625) -> (-51.49, 198.2625)
  line L237 (-64.49, 212.2625) -> (-51.49, 212.2625)
  arc A232 (-64.99, 198.7625) -> (-64.49, 198.2625) centre (-64.49, 198.7625) ccw
  arc A233 (-64.49, 212.2625) -> (-64.99, 211.7625) centre (-64.49, 211.7625) ccw
  arc A234 (-51.49, 198.2625) -> (-50.99, 198.7625) centre (-51.49, 198.7625) ccw
  arc A235 (-50.99, 211.7625) -> (-51.49, 212.2625) centre (-51.49, 211.7625) ccw
  line L238 (-64.99, 217.8125) -> (-64.99, 230.8125)
  line L239 (-50.99, 217.8125) -> (-50.99, 230.8125)
  line L240 (-64.49, 217.3125) -> (-51.49, 217.3125)
  line L241 (-64.49, 231.3125) -> (-51.49, 231.3125)
  arc A236 (-64.99, 217.8125) -> (-64.49, 217.3125) centre (-64.49, 217.8125) ccw
  arc A237 (-64.49, 231.3125) -> (-64.99, 230.8125) centre (-64.49, 230.8125) ccw
  arc A238 (-51.49, 217.3125) -> (-50.99, 217.8125) centre (-51.49, 217.8125) ccw
  arc A239 (-50.99, 230.8125) -> (-51.49, 231.3125) centre (-51.49, 230.8125) ccw
  line L242 (-64.99, 236.8625) -> (-64.99, 249.8625)
  line L243 (-50.99, 236.8625) -> (-50.99, 249.8625)
  line L244 (-64.49, 236.3625) -> (-51.49, 236.3625)
  line L245 (-64.49, 250.3625) -> (-51.49, 250.3625)
  arc A240 (-64.99, 236.8625) -> (-64.49, 236.3625) centre (-64.49, 236.8625) ccw
  arc A241 (-64.49, 250.3625) -> (-64.99, 249.8625) centre (-64.49, 249.8625) ccw
  arc A242 (-51.49, 236.3625) -> (-50.99, 236.8625) centre (-51.49, 236.8625) ccw
  arc A243 (-50.99, 249.8625) -> (-51.49, 250.3625) centre (-51.49, 249.8625) ccw
  line L246 (-64.99, 267.8188) -> (-64.99, 280.8188)
  line L247 (-50.99, 267.8188) -> (-50.99, 280.8188)
  line L248 (-64.49, 267.3188) -> (-51.49, 267.3188)
  line L249 (-64.49, 281.3188) -> (-51.49, 281.3188)
  arc A244 (-64.99, 267.8188) -> (-64.49, 267.3188) centre (-64.49, 267.8188) ccw
  arc A245 (-64.49, 281.3188) -> (-64.99, 280.8188) centre (-64.49, 280.8188) ccw
  arc A246 (-51.49, 267.3188) -> (-50.99, 267.8188) centre (-51.49, 267.8188) ccw
  arc A247 (-50.99, 280.8188) -> (-51.49, 281.3188) centre (-51.49, 280.8188) ccw
  line L250 (-63.99, 259.3808) -> (-63.99, 265.3808)
  line L251 (-48.99, 259.3808) -> (-48.99, 265.3808)
  line L252 (-63.49, 258.8808) -> (-49.49, 258.8808)
  line L253 (-63.49, 265.8808) -> (-49.49, 265.8808)
  arc A248 (-63.99, 259.3808) -> (-63.49, 258.8808) centre (-63.49, 259.3808) ccw
  arc A249 (-63.49, 265.8808) -> (-63.99, 265.3808) centre (-63.49, 265.3808) ccw
  arc A250 (-49.49, 258.8808) -> (-48.99, 259.3808) centre (-49.49, 259.3808) ccw
  arc A251 (-48.99, 265.3808) -> (-49.49, 265.8808) centre (-49.49, 265.3808) ccw
  line L254 (-63.99, 283.2568) -> (-63.99, 289.2568)
  line L255 (-48.99, 283.2568) -> (-48.99, 289.2568)
  line L256 (-63.49, 282.7568) -> (-49.49, 282.7568)
  line L257 (-63.49, 289.7568) -> (-49.49, 289.7568)
  arc A252 (-63.99, 283.2568) -> (-63.49, 282.7568) centre (-63.49, 283.2568) ccw
  arc A253 (-63.49, 289.7568) -> (-63.99, 289.2568) centre (-63.49, 289.2568) ccw
  arc A254 (-49.49, 282.7568) -> (-48.99, 283.2568) centre (-49.49, 283.2568) ccw
  arc A255 (-48.99, 289.2568) -> (-49.49, 289.7568) centre (-49.49, 289.2568) ccw
  line L258 (-45.94, 24.9313) -> (-45.94, 37.9313)
  line L259 (-31.94, 24.9313) -> (-31.94, 37.9313)
  line L260 (-45.44, 24.4313) -> (-32.44, 24.4313)
  line L261 (-45.44, 38.4313) -> (-32.44, 38.4313)
  arc A256 (-45.94, 24.9313) -> (-45.44, 24.4312) centre (-45.44, 24.9313) ccw
  arc A257 (-45.44, 38.4313) -> (-45.94, 37.9313) centre (-45.44, 37.9313) ccw
  arc A258 (-32.44, 24.4313) -> (-31.94, 24.9313) centre (-32.44, 24.9313) ccw
  arc A259 (-31.94, 37.9313) -> (-32.44, 38.4312) centre (-32.44, 37.9313) ccw
  line L262 (-44.94, 16.4933) -> (-44.94, 22.4933)
  line L263 (-29.94, 16.4933) -> (-29.94, 22.4933)
  line L264 (-44.44, 15.9933) -> (-30.44, 15.9933)
  line L265 (-44.44, 22.9933) -> (-30.44, 22.9933)
  arc A260 (-44.94, 16.4933) -> (-44.44, 15.9933) centre (-44.44, 16.4933) ccw
  arc A261 (-44.44, 22.9933) -> (-44.94, 22.4933) centre (-44.44, 22.4933) ccw
  arc A262 (-30.44, 15.9933) -> (-29.94, 16.4933) centre (-30.44, 16.4933) ccw
  arc A263 (-29.94, 22.4933) -> (-30.44, 22.9933) centre (-30.44, 22.4933) ccw
  line L266 (-44.94, 40.3693) -> (-44.94, 46.3693)
  line L267 (-29.94, 40.3693) -> (-29.94, 46.3693)
  line L268 (-44.44, 39.8693) -> (-30.44, 39.8693)
  line L269 (-44.44, 46.8693) -> (-30.44, 46.8693)
  arc A264 (-44.94, 40.3693) -> (-44.44, 39.8693) centre (-44.44, 40.3693) ccw
  arc A265 (-44.44, 46.8693) -> (-44.94, 46.3693) centre (-44.44, 46.3693) ccw
  arc A266 (-30.44, 39.8693) -> (-29.94, 40.3693) centre (-30.44, 40.3693) ccw
  arc A267 (-29.94, 46.3693) -> (-30.44, 46.8693) centre (-30.44, 46.3693) ccw
  line L270 (-45.94, 55.8875) -> (-45.94, 68.8875)
  line L271 (-31.94, 55.8875) -> (-31.94, 68.8875)
  line L272 (-45.44, 55.3875) -> (-32.44, 55.3875)
  line L273 (-45.44, 69.3875) -> (-32.44, 69.3875)
  arc A268 (-45.94, 55.8875) -> (-45.44, 55.3875) centre (-45.44, 55.8875) ccw
  arc A269 (-45.44, 69.3875) -> (-45.94, 68.8875) centre (-45.44, 68.8875) ccw
  arc A270 (-32.44, 55.3875) -> (-31.94, 55.8875) centre (-32.44, 55.8875) ccw
  arc A271 (-31.94, 68.8875) -> (-32.44, 69.3875) centre (-32.44, 68.8875) ccw
  line L274 (-45.94, 74.9375) -> (-45.94, 87.9375)
  line L275 (-31.94, 74.9375) -> (-31.94, 87.9375)
  line L276 (-45.44, 74.4375) -> (-32.44, 74.4375)
  line L277 (-45.44, 88.4375) -> (-32.44, 88.4375)
  arc A272 (-45.94, 74.9375) -> (-45.44, 74.4375) centre (-45.44, 74.9375) ccw
  arc A273 (-45.44, 88.4375) -> (-45.94, 87.9375) centre (-45.44, 87.9375) ccw
  arc A274 (-32.44, 74.4375) -> (-31.94, 74.9375) centre (-32.44, 74.9375) ccw
  arc A275 (-31.94, 87.9375) -> (-32.44, 88.4375) centre (-32.44, 87.9375) ccw
  line L278 (-45.94, 93.9875) -> (-45.94, 106.9875)
  line L279 (-31.94, 93.9875) -> (-31.94, 106.9875)
  line L280 (-45.44, 93.4875) -> (-32.44, 93.4875)
  line L281 (-45.44, 107.4875) -> (-32.44, 107.4875)
  arc A276 (-45.94, 93.9875) -> (-45.44, 93.4875) centre (-45.44, 93.9875) ccw
  arc A277 (-45.44, 107.4875) -> (-45.94, 106.9875) centre (-45.44, 106.9875) ccw
  arc A278 (-32.44, 93.4875) -> (-31.94, 93.9875) centre (-32.44, 93.9875) ccw
  arc A279 (-31.94, 106.9875) -> (-32.44, 107.4875) centre (-32.44, 106.9875) ccw
  line L282 (-45.94, 113.0375) -> (-45.94, 126.0375)
  line L283 (-31.94, 113.0375) -> (-31.94, 126.0375)
  line L284 (-45.44, 112.5375) -> (-32.44, 112.5375)
  line L285 (-45.44, 126.5375) -> (-32.44, 126.5375)
  arc A280 (-45.94, 113.0375) -> (-45.44, 112.5375) centre (-45.44, 113.0375) ccw
  arc A281 (-45.44, 126.5375) -> (-45.94, 126.0375) centre (-45.44, 126.0375) ccw
  arc A282 (-32.44, 112.5375) -> (-31.94, 113.0375) centre (-32.44, 113.0375) ccw
  arc A283 (-31.94, 126.0375) -> (-32.44, 126.5375) centre (-32.44, 126.0375) ccw
  line L286 (-45.94, 132.0875) -> (-45.94, 145.0875)
  line L287 (-31.94, 132.0875) -> (-31.94, 145.0875)
  line L288 (-45.44, 131.5875) -> (-32.44, 131.5875)
  line L289 (-45.44, 145.5875) -> (-32.44, 145.5875)
  arc A284 (-45.94, 132.0875) -> (-45.44, 131.5875) centre (-45.44, 132.0875) ccw
  arc A285 (-45.44, 145.5875) -> (-45.94, 145.0875) centre (-45.44, 145.0875) ccw
  arc A286 (-32.44, 131.5875) -> (-31.94, 132.0875) centre (-32.44, 132.0875) ccw
  arc A287 (-31.94, 145.0875) -> (-32.44, 145.5875) centre (-32.44, 145.0875) ccw
  line L290 (-45.94, 151.1375) -> (-45.94, 164.1375)
  line L291 (-31.94, 151.1375) -> (-31.94, 164.1375)
  line L292 (-45.44, 150.6375) -> (-32.44, 150.6375)
  line L293 (-45.44, 164.6375) -> (-32.44, 164.6375)
  arc A288 (-45.94, 151.1375) -> (-45.44, 150.6375) centre (-45.44, 151.1375) ccw
  arc A289 (-45.44, 164.6375) -> (-45.94, 164.1375) centre (-45.44, 164.1375) ccw
  arc A290 (-32.44, 150.6375) -> (-31.94, 151.1375) centre (-32.44, 151.1375) ccw
  arc A291 (-31.94, 164.1375) -> (-32.44, 164.6375) centre (-32.44, 164.1375) ccw
  line L294 (-45.94, 170.1875) -> (-45.94, 183.1875)
  line L295 (-31.94, 170.1875) -> (-31.94, 183.1875)
  line L296 (-45.44, 169.6875) -> (-32.44, 169.6875)
  line L297 (-45.44, 183.6875) -> (-32.44, 183.6875)
  arc A292 (-45.94, 170.1875) -> (-45.44, 169.6875) centre (-45.44, 170.1875) ccw
  arc A293 (-45.44, 183.6875) -> (-45.94, 183.1875) centre (-45.44, 183.1875) ccw
  arc A294 (-32.44, 169.6875) -> (-31.94, 170.1875) centre (-32.44, 170.1875) ccw
  arc A295 (-31.94, 183.1875) -> (-32.44, 183.6875) centre (-32.44, 183.1875) ccw
  line L298 (-45.94, 189.2375) -> (-45.94, 202.2375)
  line L299 (-31.94, 189.2375) -> (-31.94, 202.2375)
  line L300 (-45.44, 188.7375) -> (-32.44, 188.7375)
  line L301 (-45.44, 202.7375) -> (-32.44, 202.7375)
  arc A296 (-45.94, 189.2375) -> (-45.44, 188.7375) centre (-45.44, 189.2375) ccw
  arc A297 (-45.44, 202.7375) -> (-45.94, 202.2375) centre (-45.44, 202.2375) ccw
  arc A298 (-32.44, 188.7375) -> (-31.94, 189.2375) centre (-32.44, 189.2375) ccw
  arc A299 (-31.94, 202.2375) -> (-32.44, 202.7375) centre (-32.44, 202.2375) ccw
  line L302 (-45.94, 208.2875) -> (-45.94, 221.2875)
  line L303 (-31.94, 208.2875) -> (-31.94, 221.2875)
  line L304 (-45.44, 207.7875) -> (-32.44, 207.7875)
  line L305 (-45.44, 221.7875) -> (-32.44, 221.7875)
  arc A300 (-45.94, 208.2875) -> (-45.44, 207.7875) centre (-45.44, 208.2875) ccw
  arc A301 (-45.44, 221.7875) -> (-45.94, 221.2875) centre (-45.44, 221.2875) ccw
  arc A302 (-32.44, 207.7875) -> (-31.94, 208.2875) centre (-32.44, 208.2875) ccw
  arc A303 (-31.94, 221.2875) -> (-32.44, 221.7875) centre (-32.44, 221.2875) ccw
  line L306 (-45.94, 227.3375) -> (-45.94, 240.3375)
  line L307 (-31.94, 227.3375) -> (-31.94, 240.3375)
  line L308 (-45.44, 226.8375) -> (-32.44, 226.8375)
  line L309 (-45.44, 240.8375) -> (-32.44, 240.8375)
  arc A304 (-45.94, 227.3375) -> (-45.44, 226.8375) centre (-45.44, 227.3375) ccw
  arc A305 (-45.44, 240.8375) -> (-45.94, 240.3375) centre (-45.44, 240.3375) ccw
  arc A306 (-32.44, 226.8375) -> (-31.94, 227.3375) centre (-32.44, 227.3375) ccw
  arc A307 (-31.94, 240.3375) -> (-32.44, 240.8375) centre (-32.44, 240.3375) ccw
  line L310 (-45.94, 263.0563) -> (-45.94, 276.0563)
  line L311 (-31.94, 263.0563) -> (-31.94, 276.0563)
  line L312 (-45.44, 262.5563) -> (-32.44, 262.5563)
  line L313 (-45.44, 276.5563) -> (-32.44, 276.5563)
  arc A308 (-45.94, 263.0563) -> (-45.44, 262.5563) centre (-45.44, 263.0563) ccw
  arc A309 (-45.44, 276.5563) -> (-45.94, 276.0563) centre (-45.44, 276.0563) ccw
  arc A310 (-32.44, 262.5563) -> (-31.94, 263.0563) centre (-32.44, 263.0563) ccw
  arc A311 (-31.94, 276.0563) -> (-32.44, 276.5563) centre (-32.44, 276.0563) ccw
  line L314 (-44.94, 254.6183) -> (-44.94, 260.6183)
  line L315 (-29.94, 254.6183) -> (-29.94, 260.6183)
  line L316 (-44.44, 254.1183) -> (-30.44, 254.1183)
  line L317 (-44.44, 261.1183) -> (-30.44, 261.1183)
  arc A312 (-44.94, 254.6183) -> (-44.44, 254.1183) centre (-44.44, 254.6183) ccw
  arc A313 (-44.44, 261.1183) -> (-44.94, 260.6183) centre (-44.44, 260.6183) ccw
  arc A314 (-30.44, 254.1183) -> (-29.94, 254.6183) centre (-30.44, 254.6183) ccw
  arc A315 (-29.94, 260.6183) -> (-30.44, 261.1183) centre (-30.44, 260.6183) ccw
  line L318 (-44.94, 278.4943) -> (-44.94, 284.4943)
  line L319 (-29.94, 278.4943) -> (-29.94, 284.4943)
  line L320 (-44.44, 277.9943) -> (-30.44, 277.9943)
  line L321 (-44.44, 284.9943) -> (-30.44, 284.9943)
  arc A316 (-44.94, 278.4943) -> (-44.44, 277.9943) centre (-44.44, 278.4943) ccw
  arc A317 (-44.44, 284.9943) -> (-44.94, 284.4943) centre (-44.44, 284.4943) ccw
  arc A318 (-30.44, 277.9943) -> (-29.94, 278.4943) centre (-30.44, 278.4943) ccw
  arc A319 (-29.94, 284.4943) -> (-30.44, 284.9943) centre (-30.44, 284.4943) ccw
  line L322 (-45.94, 322.5875) -> (-45.94, 335.5875)
  line L323 (-31.94, 322.5875) -> (-31.94, 335.5875)
  line L324 (-45.44, 322.0875) -> (-32.44, 322.0875)
  line L325 (-45.44, 336.0875) -> (-32.44, 336.0875)
  arc A320 (-45.94, 322.5875) -> (-45.44, 322.0875) centre (-45.44, 322.5875) ccw
  arc A321 (-45.44, 336.0875) -> (-45.94, 335.5875) centre (-45.44, 335.5875) ccw
  arc A322 (-32.44, 322.0875) -> (-31.94, 322.5875) centre (-32.44, 322.5875) ccw
  arc A323 (-31.94, 335.5875) -> (-32.44, 336.0875) centre (-32.44, 335.5875) ccw
  line L326 (-26.89, 15.4063) -> (-26.89, 28.4063)
  line L327 (-12.89, 15.4063) -> (-12.89, 28.4063)
  line L328 (-26.39, 14.9063) -> (-13.39, 14.9063)
  line L329 (-26.39, 28.9063) -> (-13.39, 28.9063)
  arc A324 (-26.89, 15.4063) -> (-26.39, 14.9063) centre (-26.39, 15.4063) ccw
  arc A325 (-26.39, 28.9062) -> (-26.89, 28.4063) centre (-26.39, 28.4063) ccw
  arc A326 (-13.39, 14.9063) -> (-12.89, 15.4063) centre (-13.39, 15.4063) ccw
  arc A327 (-12.89, 28.4063) -> (-13.39, 28.9063) centre (-13.39, 28.4063) ccw
  line L330 (-26.89, 39.2188) -> (-26.89, 52.2188)
  line L331 (-12.89, 39.2188) -> (-12.89, 52.2188)
  line L332 (-26.39, 38.7188) -> (-13.39, 38.7188)
  line L333 (-26.39, 52.7188) -> (-13.39, 52.7188)
  arc A328 (-26.89, 39.2188) -> (-26.39, 38.7188) centre (-26.39, 39.2188) ccw
  arc A329 (-26.39, 52.7188) -> (-26.89, 52.2188) centre (-26.39, 52.2188) ccw
  arc A330 (-13.39, 38.7188) -> (-12.89, 39.2188) centre (-13.39, 39.2188) ccw
  arc A331 (-12.89, 52.2188) -> (-13.39, 52.7188) centre (-13.39, 52.2188) ccw
  line L334 (-26.89, 63.0313) -> (-26.89, 76.0313)
  line L335 (-12.89, 63.0313) -> (-12.89, 76.0313)
  line L336 (-26.39, 62.5313) -> (-13.39, 62.5313)
  line L337 (-26.39, 76.5313) -> (-13.39, 76.5312)
  arc A332 (-26.89, 63.0313) -> (-26.39, 62.5313) centre (-26.39, 63.0313) ccw
  arc A333 (-26.39, 76.5313) -> (-26.89, 76.0313) centre (-26.39, 76.0313) ccw
  arc A334 (-13.39, 62.5313) -> (-12.89, 63.0313) centre (-13.39, 63.0313) ccw
  arc A335 (-12.89, 76.0313) -> (-13.39, 76.5313) centre (-13.39, 76.0313) ccw
  line L338 (-26.89, 134.4688) -> (-26.89, 147.4688)